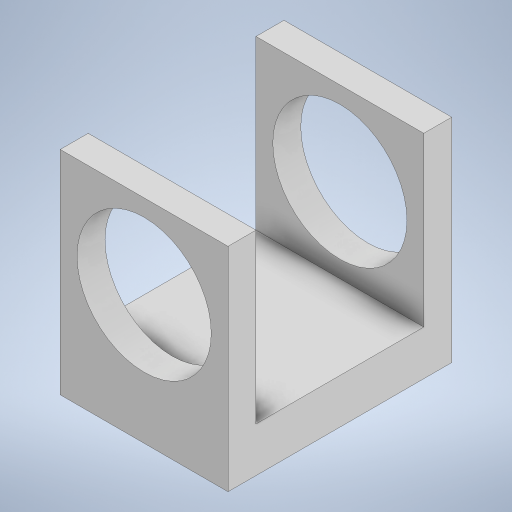
# Autodesk Inventor part: llanta_1
Saved by Autodesk Inventor 2024 (Build 280153000, 153)
## iProperties
Created: 2023-05-01
Part Number: llanta_1
Material: Generic
Document SubType Name: Modeling
Designer: Diego
Density: 1 g/cm^3
Appearance: Default
Author: Diego
Autodesk Inventor part; units mm, degrees
ref_plane "YZ Plane" through (0, 0, 0) normal (1, 0, 0) x (0, 1, 0)
ref_plane "XZ Plane" through (0, 0, 0) normal (0, 1, 0) x (-1, 0, 0)
ref_plane "XY Plane" through (0, 0, 0) normal (0, 0, 1) x (1, 0, 0)
sketch "Sketch1" plane through (0, 0, 0) normal (0, 1, 0) x (-1, 0, 0)
  line L0 (-7.5, -10) -> (7.5, -10)
  line L1 (7.5, -10) -> (7.5, 10)
  line L2 (7.5, 10) -> (-7.5, 10)
  line L3 (-7.5, 10) -> (-7.5, -10)
  line L4 (-7.5, -10) -> (7.5, 10) construction
  line L5 (7.5, -10) -> (-7.5, 10) construction
  point P0 (0, 0)
  dimension "d0" = 15
  dimension "d1" = 20
  constraints: 12 end point, 2 midpoint, 2 parallel, 1 horizontal, 1 perpendicular
  measures "d0" distance of L2.end L1.end
  measures "d1" distance of L1.end L0.end
extrude "Extrusion1" add sketch "Sketch1" along normal blind 4
sketch "Sketch2" plane through (0, 4, 0) normal (0, 1, 0) x (1, 0, 0)
  line L0 (-7.5, 10) -> (-7.5, -10) projected
  line L1 (7.5, -10) -> (7.5, 10) projected
  line L2 (-7.5, 10) -> (7.5, 10)
  line L3 (7.5, 10) -> (7.5, 7.5)
  line L4 (7.5, 7.5) -> (-7.5, 7.5)
  line L5 (-7.5, 7.5) -> (-7.5, 10)
  line L6 (7.5, 0) -> (0, 0) construction
  line L7 (-7.5, -10) -> (-7.5, 10)
  line L8 (7.5, 10) -> (7.5, -10)
  line L9 (-7.5, -10) -> (7.5, -10)
  line L10 (7.5, -7.5) -> (-7.5, -7.5)
  dimension "d4" = 2.5
  constraints: 18 end point, 7 symmetric about line, 2 horizontal, 2 parallel, 2 point on line, 1 midpoint, 1 perpendicular
  measures "d4" distance of L2.end L3.end
extrude "Extrusion2" add sketch "Sketch2" along normal blind 15 contours L2 L1 L4 L0 | L10 L1 L9 L0
sketch "Sketch3" plane through (-7.5, 0, 10) normal (0, 0, 1) x (1, 0, 0)
  line L0 (15, 19) -> (0, 19) construction
  line L1 (7.5, 19) -> (7.5, 0) construction
  line L2 (7.5, 0) -> (7.5, 4) construction
  line L3 (0, 0) -> (0, 19) construction
  line L4 (15, 4) -> (0, 4) construction
  line L5 (0, 4) -> (15, 4) construction
  line L6 (0, 19) -> (15, 4) construction
  line L7 (15, 19) -> (0, 4) construction
  circle A0 centre (7.5, 11.5) radius 6
  dimension "d7" = 4
  dimension "d8" = 12
  constraints: 10 end point, 2 midpoint, 2 point on line, 1 centre point, 1 horizontal, 1 perpendicular, 1 vertical
  measures "d7" distance of L1.end L2.end
  measures "d8" diameter of A0
extrude "Extrusion3" cut sketch "Sketch3" against normal blind 23.5
body "Solid1"
